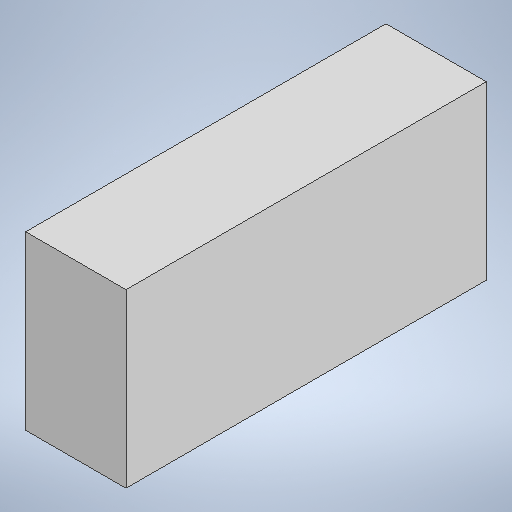
# Autodesk Inventor part: Lipo Battery 9500mAh 29.6V
Saved by Autodesk Inventor 2025.1 (Build 291241000, 241)
## iProperties
Created: 2025-04-08
Part Number: Lipo Battery 9500mAh 29.6V
Material: Типовые
Document SubType Name: Modeling
Designer: Root
Mass: 1450 g
Surface Area: 550.48 cm^2
Volume: 724.416 cm^3
Density: 2.00161 g/cm^3
Appearance: По умолчанию
Author: Root
Autodesk Inventor part; units mm, degrees
ref_plane "YZ Plane" through (0, 0, 0) normal (1, 0, 0) x (0, 1, 0)
ref_plane "XZ Plane" through (0, 0, 0) normal (0, 1, 0) x (-1, 0, 0)
ref_plane "XY Plane" through (0, 0, 0) normal (0, 0, 1) x (1, 0, 0)
sketch "Эскиз1" plane through (0, 0, 0) normal (0, 1, 0) x (-1, 0, 0)
  line L0 (-24.5, -88) -> (24.5, -88)
  line L1 (24.5, -88) -> (24.5, 88)
  line L2 (24.5, 88) -> (-24.5, 88)
  line L3 (-24.5, 88) -> (-24.5, -88)
  line L4 (-24.5, -88) -> (24.5, 88) construction
  line L5 (24.5, -88) -> (-24.5, 88) construction
  point P0 (0, 0)
  dimension "d0" = 49
  dimension "d1" = 176
  constraints: 12 end point, 2 midpoint, 2 parallel, 1 horizontal, 1 perpendicular
  measures "d0" distance of L2.end L1.end
  measures "d1" distance of L1.end L0.end
extrude "Выдавливание1" add sketch "Эскиз1" along normal mid plane 84
